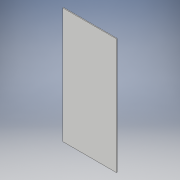
# Autodesk Inventor part: arm_enclosure_door_panel
Saved by Autodesk Inventor 2019 (Build 230136000, 136)
## iProperties
Created: 2018-07-20
Part Number: arm_enclosure_door_panel
Material: Generic
Document SubType Name: Modeling
Designer: Brian
Density: 1 g/cm^3
Appearance: Default
Author: Brian
Autodesk Inventor part; units mm, degrees
ref_plane "YZ Plane" through (0, 0, 0) normal (1, 0, 0) x (0, 1, 0)
ref_plane "XZ Plane" through (0, 0, 0) normal (0, 1, 0) x (-1, 0, 0)
ref_plane "XY Plane" through (0, 0, 0) normal (0, 0, 1) x (1, 0, 0)
sketch "Sketch1" plane through (0, 0, 0) normal (0, 0, 1) x (1, 0, 0)
  line L0 (0, 0) -> (419.1, 0)
  line L1 (419.1, 0) -> (419.1, 901.7)
  line L2 (419.1, 901.7) -> (0, 901.7)
  line L3 (0, 901.7) -> (0, 0)
  dimension "d0" = 419.1
  dimension "d1" = 901.7
  constraints: 8 end point, 2 parallel, 1 horizontal, 1 perpendicular
  measures "d0" distance of L2.end L1.end
  measures "d1" distance of L1.end L0.end
extrude "Extrusion1" add sketch "Sketch1" along normal blind 6.35
body "Solid1"
